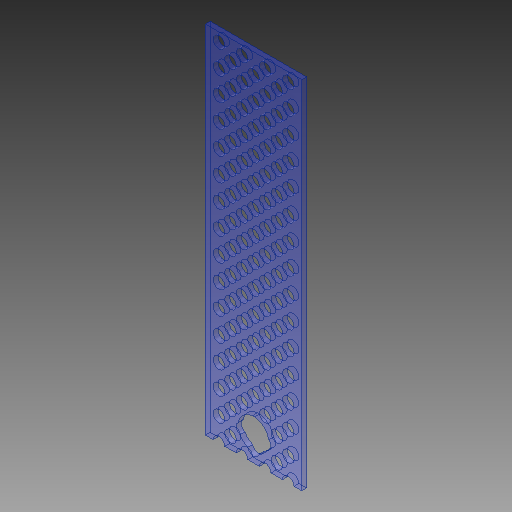
# Autodesk Inventor part: tank_front
Saved by Autodesk Inventor 2018.1 (Build 221171000, 171)
## iProperties
Created: 2017-07-30
Part Number: tank_front
Material: PVC-Piping
Document SubType Name: Modeling
Designer: Tom
Density: 1.4 g/cm^3
Appearance: Clear - Blue
Mass: 123.583 g
Surface Area: 669.185 cm^2
Volume: 88.2739 cm^3
Author: Tom
Autodesk Inventor part; units mm, degrees
ref_plane "YZ Plane" through (0, 0, 0) normal (1, 0, 0) x (0, 1, 0)
ref_plane "XZ Plane" through (0, 0, 0) normal (0, 1, 0) x (-1, 0, 0)
ref_plane "XY Plane" through (0, 0, 0) normal (0, 0, 1) x (1, 0, 0)
sketch "Sketch1" plane through (0, 0, 0) normal (0, 0, 1) x (1, 0, 0)
  line L0 (0, 0) -> (100, 0)
  line L1 (100, 0) -> (100, 370)
  line L2 (100, 370) -> (0, 370)
  line L3 (0, 370) -> (0, 0)
  dimension "d0" = 100
  dimension "d1" = 370
  constraints: 8 end point, 2 parallel, 1 horizontal, 1 perpendicular
  measures "d0" distance of L2.end L1.end
  measures "d1" distance of L1.end L0.end
extrude "Extrusion1" add sketch "Sketch1" along normal blind 5
sketch "Sketch2" plane through (0, 0, 5) normal (0, 0, 1) x (1, 0, 0)
  circle A0 centre (13.9375, 0) radius 6
  line L0 (0, 370) -> (0, 0) projected
  line L1 (0, 0) -> (100, 0) projected
  circle A1 centre (25.9583, 12.0208) radius 6
  circle A2 centre (13.9375, 24.0416) radius 6
  circle A3 centre (13.9375, 48.0833) radius 6
  circle A4 centre (13.9375, 72.1249) radius 6
  circle A5 centre (13.9375, 96.1665) radius 6
  circle A6 centre (13.9375, 120.2082) radius 6
  circle A7 centre (13.9375, 144.2498) radius 6
  circle A8 centre (13.9375, 168.2914) radius 6
  circle A9 centre (13.9375, 192.333) radius 6
  circle A10 centre (13.9375, 216.3747) radius 6
  circle A11 centre (13.9375, 240.4163) radius 6
  circle A12 centre (13.9375, 264.4579) radius 6
  circle A13 centre (13.9375, 288.4996) radius 6
  circle A14 centre (13.9375, 312.5412) radius 6
  circle A15 centre (13.9375, 336.5828) radius 6
  circle A16 centre (37.9791, 0) radius 6
  circle A17 centre (37.9791, 24.0416) radius 6
  circle A18 centre (37.9791, 48.0833) radius 6
  circle A19 centre (37.9791, 72.1249) radius 6
  circle A20 centre (37.9791, 96.1665) radius 6
  circle A21 centre (37.9791, 120.2082) radius 6
  circle A22 centre (37.9791, 144.2498) radius 6
  circle A23 centre (37.9791, 168.2914) radius 6
  circle A24 centre (37.9791, 192.333) radius 6
  circle A25 centre (37.9791, 216.3747) radius 6
  circle A26 centre (37.9791, 240.4163) radius 6
  circle A27 centre (37.9791, 264.4579) radius 6
  circle A28 centre (37.9791, 288.4996) radius 6
  circle A29 centre (37.9791, 312.5412) radius 6
  circle A30 centre (37.9791, 336.5828) radius 6
  circle A31 centre (62.0208, 0) radius 6
  circle A32 centre (62.0208, 24.0416) radius 6
  circle A33 centre (62.0208, 48.0833) radius 6
  circle A34 centre (62.0208, 72.1249) radius 6
  circle A35 centre (62.0208, 96.1665) radius 6
  circle A36 centre (62.0208, 120.2082) radius 6
  circle A37 centre (62.0208, 144.2498) radius 6
  circle A38 centre (62.0208, 168.2914) radius 6
  circle A39 centre (62.0208, 192.333) radius 6
  circle A40 centre (62.0208, 216.3747) radius 6
  circle A41 centre (62.0208, 240.4163) radius 6
  circle A42 centre (62.0208, 264.4579) radius 6
  circle A43 centre (62.0208, 288.4996) radius 6
  circle A44 centre (62.0208, 312.5412) radius 6
  circle A45 centre (62.0208, 336.5828) radius 6
  circle A46 centre (86.0624, 0) radius 6
  circle A47 centre (86.0624, 24.0416) radius 6
  circle A48 centre (86.0624, 48.0833) radius 6
  circle A49 centre (86.0624, 72.1249) radius 6
  circle A50 centre (86.0624, 96.1665) radius 6
  circle A51 centre (86.0624, 120.2082) radius 6
  circle A52 centre (86.0624, 144.2498) radius 6
  circle A53 centre (86.0624, 168.2914) radius 6
  circle A54 centre (86.0624, 192.333) radius 6
  circle A55 centre (86.0624, 216.3747) radius 6
  circle A56 centre (86.0624, 240.4163) radius 6
  circle A57 centre (86.0624, 264.4579) radius 6
  circle A58 centre (86.0624, 288.4996) radius 6
  circle A59 centre (86.0624, 312.5412) radius 6
  circle A60 centre (86.0624, 336.5828) radius 6
  circle A61 centre (25.9583, 36.0624) radius 6
  circle A62 centre (25.9583, 60.1041) radius 6
  circle A63 centre (25.9583, 84.1457) radius 6
  circle A64 centre (25.9583, 108.1873) radius 6
  circle A65 centre (25.9583, 132.229) radius 6
  circle A66 centre (25.9583, 156.2706) radius 6
  circle A67 centre (25.9583, 180.3122) radius 6
  circle A68 centre (25.9583, 204.3539) radius 6
  circle A69 centre (25.9583, 228.3955) radius 6
  circle A70 centre (25.9583, 252.4371) radius 6
  circle A71 centre (25.9583, 276.4788) radius 6
  circle A72 centre (25.9583, 300.5204) radius 6
  circle A73 centre (25.9583, 324.562) radius 6
  circle A74 centre (25.9583, 348.6036) radius 6
  circle A75 centre (49.9999, 12.0208) radius 6
  circle A76 centre (49.9999, 36.0624) radius 6
  circle A77 centre (49.9999, 60.1041) radius 6
  circle A78 centre (49.9999, 84.1457) radius 6
  circle A79 centre (49.9999, 108.1873) radius 6
  circle A80 centre (49.9999, 132.229) radius 6
  circle A81 centre (49.9999, 156.2706) radius 6
  circle A82 centre (49.9999, 180.3122) radius 6
  circle A83 centre (49.9999, 204.3539) radius 6
  circle A84 centre (49.9999, 228.3955) radius 6
  circle A85 centre (49.9999, 252.4371) radius 6
  circle A86 centre (49.9999, 276.4788) radius 6
  circle A87 centre (49.9999, 300.5204) radius 6
  circle A88 centre (49.9999, 324.562) radius 6
  circle A89 centre (49.9999, 348.6036) radius 6
  circle A90 centre (74.0416, 12.0208) radius 6
  circle A91 centre (74.0416, 36.0624) radius 6
  circle A92 centre (74.0416, 60.1041) radius 6
  circle A93 centre (74.0416, 84.1457) radius 6
  circle A94 centre (74.0416, 108.1873) radius 6
  circle A95 centre (74.0416, 132.229) radius 6
  circle A96 centre (74.0416, 156.2706) radius 6
  circle A97 centre (74.0416, 180.3122) radius 6
  circle A98 centre (74.0416, 204.3539) radius 6
  circle A99 centre (74.0416, 228.3955) radius 6
  circle A100 centre (74.0416, 252.4371) radius 6
  circle A101 centre (74.0416, 276.4788) radius 6
  circle A102 centre (74.0416, 300.5204) radius 6
  circle A103 centre (74.0416, 324.562) radius 6
  circle A104 centre (74.0416, 348.6036) radius 6
  line L2 (100, 0) -> (100, 370) projected
  circle A105 centre (13.9375, 360.6245) radius 6
  circle A106 centre (37.9791, 360.6245) radius 6
  circle A107 centre (62.0208, 360.6245) radius 6
  circle A108 centre (86.0624, 360.6245) radius 6
  dimension "d24" = 13.9375
  dimension "d25" = 0
  dimension "d26" = 12.0208
  dimension "d27" = 12.0208
  dimension "d34" = 24.0416
  dimension "d37" = 24.0416
  dimension "d42" = 24.0416
  dimension "d45" = 24.0416
  dimension "d48" = 13.9376
  constraints: 109 centre point, 2 horizontal, 2 vertical, 214 other
  measures "d24" distance from line of A0.centre L0
  measures "d25" distance from line of L1 A0.centre
  measures "d26" horizontal distance of A1.centre A0.centre
  measures "d27" horizontal distance of A0.centre A1.centre
  measures "d34" distance of A0.centre A2.centre
  measures "d37" distance of A0.centre A16.centre
  measures "d42" distance of A1.centre A61.centre
  measures "d45" distance of A1.centre A75.centre
  measures "d48" distance from line of L2 A46.centre
sketch "Sketch3" plane through (0, 0, 5) normal (0, 0, 1) x (1, 0, 0)
  circle A0 centre (50, 26) radius 16 projected
  point P0 (0, 0)
extrude "Extrusion3" cut sketch "Sketch3" against normal blind 5
extrude "Extrusion4" cut sketch "Sketch2" against normal blind 5
equation "\"d0\" = tankw"
equation "\"d1\" = tankh"
equation "\"d2\" = pvct"
equation "\"d24\" = sidedist"
equation "\"d26\" = gratespacing"
equation "\"d27\" = gratespacing"
equation "\"d34\" = 2 * gratespacing"
equation "\"d37\" = 2 * gratespacing"
equation "\"d42\" = 2 * gratespacing"
equation "\"d45\" = 2 * gratespacing"
equation "\"d30\" = pvct"
equation "\"d49\" = pvct"
equation "\"lcsd\" = 19.05"
equation "\"lcwd1\" = 25"
equation "\"lcwd2\" = 34"
equation "\"lch1\" = 39"
equation "\"lcwd3\" = 43"
equation "\"dia1\" = 6"
equation "\"td\" = 18"
equation "\"bhh\" = 6"
equation "\"sw\" = 25"
equation "\"sh\" = 31"
equation "\"spacert\" = 2"
equation "\"pvct\" = 5"
equation "\"tankw\" = 100"
equation "\"tankh\" = 370"
equation "\"tankl\" = 379"
equation "\"dia3\" = 8"
equation "\"dia4\" = 11"
equation "\"play\" = 9"
equation "\"holeh\" = 26"
equation "\"surroundt\" = 5"
equation "\"slack\" = 0.5"
equation "\"play2\" = 3"
equation "\"diaoverflow\" = 25"
equation "\"diacucl\" = 32"
equation "\"diawater\" = 25"
equation "\"diaph\" = 32"
equation "\"diaair\" = 32"
equation "\"diasurroundhole\" = 42"
equation "\"diagrate\" = 12"
equation "\"gratespacing\" = 12.02082"
equation "\"sidedist\" = 13.9375"
equation "\"bottomdist\" = 9.6355"
equation "\"diahcl\" = 32"
equation "\"bracketwtop\" = 6"
equation "\"bracketwbottom\" = 6"
equation "\"nett\" = 1"
equation "\"nethole\" = 16"
equation "\"nettop\" = 7"
equation "\"netside\" = 3.5"
equation "\"netholespacing\" = 2"
equation "\"diaetape\" = 32"
body "Solid1"
